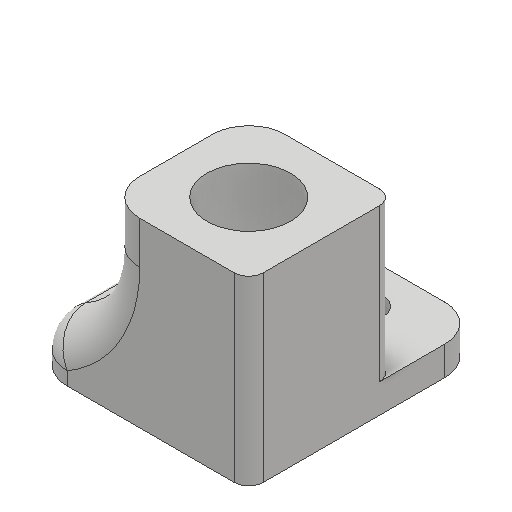
# Autodesk Inventor part: 3DP_ABS_Feet
Saved by Autodesk Inventor 2026.1 (Build 301233000, 233)
## iProperties
Created: 2017-05-24
Part Number: 3DP_ABS_Feet
Material: Ogólny
Document SubType Name: Modeling
Designer: Andrzej
Density: 1 g/cm^3
Appearance: Domyślna
Mass: 9.96617 g
Surface Area: 44.0355 cm^2
Volume: 9.96617 cm^3
Author: Andrzej
Autodesk Inventor part; units mm, degrees
ref_plane "YZ Plane" through (0, 0, 0) normal (1, 0, 0) x (0, 1, 0)
ref_plane "XZ Plane" through (0, 0, 0) normal (0, 1, 0) x (-1, 0, 0)
ref_plane "XY Plane" through (0, 0, 0) normal (0, 0, 1) x (1, 0, 0)
sketch "Szkic1" plane through (0, 0, 0) normal (0, 0, 1) x (1, 0, 0)
  line L0 (-16.0043, 3.0513) -> (-16.0043, -16.9487)
  line L1 (-16.0043, -16.9487) -> (13.9957, -16.9487)
  line L2 (13.9957, -16.9487) -> (13.9957, 15.0513)
  line L3 (13.9957, 15.0513) -> (-6.0043, 15.0513)
  line L4 (-6.0043, 15.0513) -> (-6.0043, 3.0513)
  line L5 (-6.0043, 3.0513) -> (-16.0043, 3.0513)
  point P0 (0, 0)
  dimension "d0" = 20
  dimension "d1" = 30
  dimension "d2" = 32
  dimension "d3" = 20
  constraints: 12 end point, 4 perpendicular, 1 horizontal, 1 vertical
  measures "d0" distance of L0.start L0.end
  measures "d1" distance of L0.end L1.end
  measures "d2" distance of L1.end L2.end
  measures "d3" distance of L2.end L3.end
extrude "Wyciągnięcie proste1" add sketch "Szkic1" along normal blind 4
sketch "Szkic2" plane through (0, 0, 4) normal (0, 0, 1) x (1, 0, 0)
  line L0 (-16.0043, 3.0513) -> (-16.0043, -16.9487) projected
  line L1 (-16.0043, -16.9487) -> (13.9957, -16.9487) projected
  line L2 (13.9957, -16.9487) -> (13.9957, 15.0513) projected
  line L3 (13.9957, 15.0513) -> (-6.0043, 15.0513) projected
  line L4 (-6.0043, 15.0513) -> (-6.0043, 3.0513) projected
  line L5 (-6.0043, 3.0513) -> (-16.0043, 3.0513) projected
  line L6 (-6.0043, 15.0513) -> (-6.0043, 3.0513) projected
  line L7 (-6.0043, 3.0513) -> (-16.0043, 3.0513) projected
  line L8 (-6.0043, 3.0513) -> (13.9957, 3.0513)
  line L9 (-6.0043, 3.0513) -> (-6.0043, -16.9487)
  line L10 (-16.0043, -16.9487) -> (13.9957, -16.9487) projected
  point P0 (0, 0)
  constraints: 4 end point, 2 perpendicular, 2 point on line
extrude "Wyciągnięcie proste2" add sketch "Szkic2" along normal blind 1 contours L5 L9 L1 L0
extrude "Wyciągnięcie proste3" add sketch "Szkic2" along normal blind 21 contours L8 L2 L1 L9
fillet "Zaokrąglenie1" radius 15 1 edges at (-6.0043, -6.9487, 5)
fillet "Zaokrąglenie1" radius 5 1 edges at (-16.0043, -6.9487, 5)
fillet "Zaokrąglenie2" radius 5 8 edges at (-15.3344, -16.9487, 4.3216) (-16.0043, -16.9487, 0.9108) (-6.0043, -16.9487, 22.0711) (-8.0139, -16.9487, 11.6421) (-15.3344, 3.0513, 4.3216) (-16.0043, 3.0513, 0.9108) (-6.0043, 3.0513, 22.0711) (-8.0139, 3.0513, 11.6421)
fillet "Zaokrąglenie2" radius 2 2 edges at (13.9957, 3.0513, 14.5) (13.9957, -16.9487, 12.5)
fillet "Zaokrąglenie2" radius 5 2 edges at (-6.0043, 15.0513, 2) (13.9957, 15.0513, 2)
sketch "Szkic3" plane through (0, 0, 25) normal (0, 0, 1) x (1, 0, 0)
  arc A0 (11.9957, -16.9487) -> (13.9957, -14.9487) centre (11.9957, -14.9487) ccw projected
  line L0 (13.9957, -14.9487) -> (13.9957, 1.0513) projected
  arc A1 (13.9957, 1.0513) -> (11.9957, 3.0513) centre (11.9957, 1.0513) ccw projected
  line L1 (11.9957, 3.0513) -> (-1.0043, 3.0513) projected
  arc A2 (-1.0043, 3.0513) -> (-6.0043, -1.9487) centre (-1.0043, -1.9487) ccw projected
  line L2 (-6.0043, -1.9487) -> (-6.0043, -11.9487) projected
  arc A3 (-6.0043, -11.9487) -> (-1.0043, -16.9487) centre (-1.0043, -11.9487) ccw projected
  line L3 (-1.0043, -16.9487) -> (11.9957, -16.9487) projected
  circle A4 centre (3.9957, -6.9487) radius 5.75
  point P0 (0, 0)
  dimension "d15" = 20
  dimension "d16" = 10
  dimension "d17" = 10
  dimension "d18" = 11.5
  constraints: 1 centre point, 1 coincident
  measures "d15" distance between parallel lines of L2 L0
  measures "d16" distance from line of L0 point (3.996, -6.949)
  measures "d17" distance from line of L3 point (3.996, -6.949)
  measures "d18" diameter of A4
extrude "Wyciągnięcie proste4" cut sketch "Szkic3" against normal blind 21 contours A4
sketch "Szkic4" plane through (0, 0, 4) normal (0, 0, 1) x (1, 0, 0)
  circle A0 centre (3.9957, -6.9487) radius 5.75 projected
  arc A1 (13.9957, 10.0513) -> (8.9957, 15.0513) centre (8.9957, 10.0513) ccw projected
  line L0 (8.9957, 15.0513) -> (-1.0043, 15.0513) projected
  arc A2 (-1.0043, 15.0513) -> (-6.0043, 10.0513) centre (-1.0043, 10.0513) ccw projected
  line L1 (-6.0043, 10.0513) -> (-6.0043, 3.0513) projected
  line L2 (-6.0043, 3.0513) -> (11.9957, 3.0513) projected
  arc A3 (13.9957, 1.0513) -> (11.9957, 3.0513) centre (11.9957, 1.0513) ccw projected
  line L3 (13.9957, 1.0513) -> (13.9957, 10.0513) projected
  point P0 (0, 0)
  point P1 (3.9957, 9.0513)
  dimension "d21" = 10
  dimension "d22" = 12
  dimension "d23" = 6
  constraints: 1 coincident
  measures "d21" distance from line of L1 point (3.996, 9.051)
  measures "d22" distance between parallel lines of L0 L2
  measures "d23" distance from line of L0 point (3.996, 9.051)
hole "Otwór1" at (3.9957, -6.9487, 4) at (3.9957, 9.0513, 4) direction (0, 0, -1) diameter 5 depth 8
equation "\"d23\" = 0.5 * d22"
